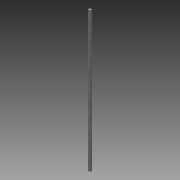
# Autodesk Inventor part: Aluminium Rod
Saved by Autodesk Inventor 2015 SP1 (Build 190203100, 203)
## iProperties
Created: 2014-09-22
Part Number: Aluminium Rod
Material: Generic
Document SubType Name: Modeling
Designer: I Rabey
Density: 1 g/cm^3
Appearance: Default
Author: I Rabey
Autodesk Inventor part; units mm, degrees
ref_plane "YZ Plane" through (0, 0, 0) normal (1, 0, 0) x (0, 1, 0)
ref_plane "XZ Plane" through (0, 0, 0) normal (0, 1, 0) x (-1, 0, 0)
ref_plane "XY Plane" through (0, 0, 0) normal (0, 0, 1) x (1, 0, 0)
sketch "Sketch1" plane through (0, 0, 0) normal (0, 1, 0) x (-1, 0, 0)
  line L0 (-6.35, 6.35) -> (6.35, 6.35)
  line L1 (6.35, 6.35) -> (6.35, -6.35)
  line L2 (6.35, -6.35) -> (-6.35, -6.35)
  line L3 (-6.35, -6.35) -> (-6.35, 6.35)
  line L4 (-6.35, 6.35) -> (6.35, -6.35) construction
  line L5 (6.35, 6.35) -> (-6.35, -6.35) construction
  point P0 (0, 0)
  dimension "d0" = 12.7
  dimension "d1" = 12.7
  constraints: 12 end point, 2 midpoint, 2 parallel, 1 horizontal, 1 perpendicular
  measures "d0" distance of L1.end L2.end
  measures "d1" distance of L0.end L1.end
extrude "Extrusion1" add sketch "Sketch1" along normal blind 900
sketch "Sketch25" plane through (6.35, 0, 6.35) normal (0, 0, 1) x (1, 0, 0)
  circle A0 centre (-6.35, 875) radius 2.5
  line L0 (-12.7, 900) -> (0, 900) projected
  line L1 (0, 0) -> (0, 900) projected
  circle A1 centre (-6.35, 857) radius 2.5
  circle A2 centre (-6.35, 705) radius 2.5
  circle A3 centre (-6.35, 578) radius 2.5
  circle A4 centre (-6.35, 451) radius 2.5
  circle A5 centre (-6.35, 324) radius 2.5
  circle A6 centre (-6.35, 194) radius 2.5
  line L2 (0, 0) -> (-12.7, 0) projected
  point P0 (-6.35, 0)
  dimension "d197" = 5
  dimension "d198" = 25
  dimension "d199" = 6.35
  dimension "d200" = 5
  dimension "d201" = 18
  dimension "d202" = 6.35
  dimension "d210" = 5
  dimension "d211" = 152
  dimension "d212" = 6.35
  dimension "d213" = 5
  dimension "d214" = 127
  dimension "d215" = 5
  dimension "d216" = 127
  dimension "d217" = 5
  dimension "d218" = 127
  dimension "d219" = 5
  dimension "d220" = 130
  constraints: 7 centre point
  measures "d197" diameter of A0
  measures "d198" distance from line of L0 A0.centre
  measures "d199" distance from line of L1 A0.centre
  measures "d200" diameter of A1
  measures "d201" distance of A1.centre A0.centre
  measures "d202" distance from line of L1 A1.centre
  measures "d210" diameter of A2
  measures "d211" distance of A2.centre A1.centre
  measures "d212" distance from line of L1 A2.centre
  measures "d213" diameter of A3
  measures "d214" distance of A2.centre A3.centre
  measures "d215" diameter of A4
  measures "d216" distance of A4.centre A3.centre
  measures "d217" diameter of A5
  measures "d218" distance of A4.centre A5.centre
  measures "d219" diameter of A6
  measures "d220" distance of A6.centre A5.centre
hole "Hole23" at (0, 875, 6.35) at (0, 857, 6.35) at (0, 705, 6.35) at (0, 578, 6.35) at (0, 451, 6.35) at (0, 324, 6.35) at (0, 194, 6.35) direction (0, 0, -1) diameter 5 end through all
sketch "Sketch26" plane through (6.35, 0, -6.35) normal (1, 0, 0) x (0, 0, -1)
  circle A0 centre (-6.35, 883.5) radius 2.5
  line L0 (-12.7, 900) -> (0, 900) projected
  circle A1 centre (-6.35, 858.1) radius 2.5
  circle A2 centre (-6.35, 781.9) radius 2.5
  circle A3 centre (-6.35, 654.9) radius 2.5
  circle A4 centre (-6.35, 527.9) radius 2.5
  circle A5 centre (-6.35, 400.9) radius 2.5
  circle A6 centre (-6.35, 273.9) radius 2.5
  circle A7 centre (-6.35, 255.8152) radius 2.5
  circle A8 centre (-6.35, 230.4152) radius 2.5
  point P0 (-6.35, 0)
  dimension "d231" = 5
  dimension "d232" = 16.5
  dimension "d233" = 5
  dimension "d234" = 25.4
  dimension "d235" = 5
  dimension "d236" = 76.2
  dimension "d237" = 5
  dimension "d238" = 127
  dimension "d239" = 5
  dimension "d240" = 127
  dimension "d241" = 5
  dimension "d242" = 127
  dimension "d243" = 5
  dimension "d244" = 127
  dimension "d245" = 5
  dimension "d246" = 18.0848
  dimension "d247" = 5
  dimension "d248" = 25.4
  constraints: 9 centre point
  measures "d231" diameter of A0
  measures "d232" distance from line of L0 A0.centre
  measures "d233" diameter of A1
  measures "d234" distance of A1.centre A0.centre
  measures "d235" diameter of A2
  measures "d236" distance of A2.centre A1.centre
  measures "d237" diameter of A3
  measures "d238" distance of A3.centre A2.centre
  measures "d239" diameter of A4
  measures "d240" distance of A3.centre A4.centre
  measures "d241" diameter of A5
  measures "d242" distance of A5.centre A4.centre
  measures "d243" diameter of A6
  measures "d244" distance of A6.centre A5.centre
  measures "d245" diameter of A7
  measures "d246" distance of A6.centre A7.centre
  measures "d247" diameter of A8
  measures "d248" distance of A8.centre A7.centre
hole "Hole24" at (6.35, 883.5, 0) at (6.35, 858.1, 0) at (6.35, 781.9, 0) at (6.35, 654.9, 0) at (6.35, 527.9, 0) at (6.35, 400.9, 0) at (6.35, 273.9, 0) at (6.35, 255.8152, 0) at (6.35, 230.4152, 0) direction (-1, 0, 0) diameter 5 end through all
body "Solid1"
